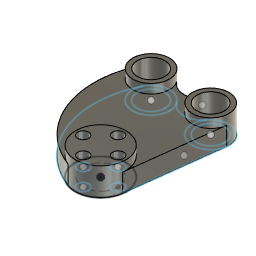
ex81 (Autodesk Fusion 360 design; units mm, degrees)
Autodesk Fusion 360 part; units mm, degrees
sketch "Sketch1" plane through (0, 0, 0) normal (0, 0, 1) x (1, 0, 0)
  circle A0 centre (0, 0) radius 27.5
  circle A1 centre (0, 0) radius 19 construction
  circle A2 centre (19, 0) radius 6
  circle A3 centre (0, 19) radius 6
  circle A4 centre (-19, 0) radius 6
  circle A5 centre (0, -19) radius 6
  circle A6 centre (-45, 100) radius 15
  circle A7 centre (-45, 100) radius 20
  circle A8 centre (20, 100) radius 15
  circle A9 centre (20, 100) radius 20
  arc A10 (-28.75, 111.6592) -> (3.75, 111.6592) centre (-12.5, 123.3184) ccw
  arc A11 (-62.9834, 108.752) -> (-9.8045, -25.6928) centre (25.1352, 65.8671) ccw
  line L0 (39.847, 97.5306) -> (27.2896, -3.3954)
  dimension "d1" = 55
  dimension "d2" = 38
  dimension "d3" = 12
  dimension "d5" = 360
  dimension "d8" = 30
  dimension "d9" = 40
  dimension "d10" = 65
  dimension "d11" = 30
  dimension "d12" = 40
  dimension "d13" = 40
  dimension "d14" = 196
  constraint coincident A0.centre A1.centre
  constraint coincident A1 A2.centre
  constraint concentric A6 A7
  constraint concentric A8 A9
  constraint tangent A7 A10
  constraint tangent A9 A10
  constraint coincident A9 A10.end
  constraint coincident A7 A10.start
  constraint tangent A7 A11
  constraint tangent A0 A11
  constraint coincident A0 A11.end
  constraint coincident A7 A11.start
  constraint tangent A9 L0
  constraint tangent A0 L0
  constraint coincident A0 L0.end
  constraint coincident A9 L0.start
  measures "d1" diameter of A0
  measures "d2" diameter of A1
  measures "d3" diameter of A2
  measures "d8" diameter of A6
  measures "d9" diameter of A7
  measures "d10" distance of A6.centre A8.centre
  measures "d11" diameter of A8
  measures "d12" diameter of A9
  measures "d13" diameter of A10
  measures "d14" diameter of A11
extrude "Extrude1" add sketch "Sketch1" along normal blind 30 contours A7 | A9 makes body 1 at (39.9006, 101.9914, 20) makes body 2 at (-25.0994, 101.9914, 20)
extrude "Extrude2" add sketch "Sketch1" along normal blind 20 contours A0 A7 A9 A10 A11 L0 bodies 1 2
extrude "Extrude3" add sketch "Sketch1" along normal blind 30 contours A0 bodies 1
